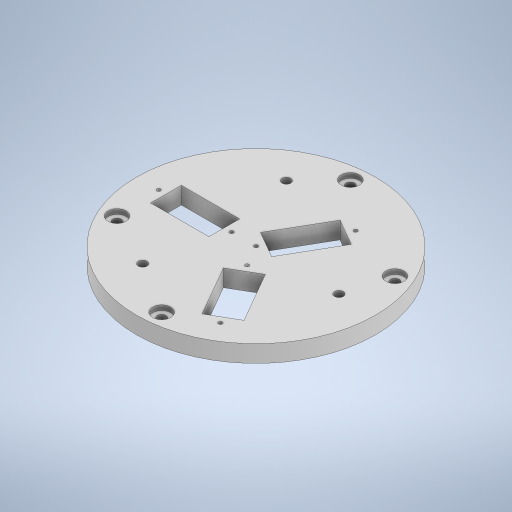
# Autodesk Inventor part: Servo Mounts
Saved by Autodesk Inventor 2023 (Build 270158000, 158)
## iProperties
Created: 2023-07-20
Part Number: Servo Mounts
Material: Generic
Document SubType Name: Modeling
Designer: campstudent
Density: 1 g/cm^3
Appearance: Default
Author: campstudent
Autodesk Inventor part; units mm, degrees
ref_plane "YZ Plane" through (0, 0, 0) normal (1, 0, 0) x (0, 1, 0)
ref_plane "XZ Plane" through (0, 0, 0) normal (0, 1, 0) x (-1, 0, 0)
ref_plane "XY Plane" through (0, 0, 0) normal (0, 0, 1) x (1, 0, 0)
sketch "Sketch1" plane through (0, 0, 0) normal (0, 1, 0) x (-1, 0, 0)
  circle A0 centre (0, 0) radius 45 construction
  line L0 (36.9, 6.3) -> (13, 6.3)
  line L1 (13, 6.3) -> (13, -6.3)
  line L2 (13, -6.3) -> (36.9, -6.3)
  line L3 (36.9, -6.3) -> (36.9, 6.3)
  line L4 (-12.994, 35.1063) -> (-23.906, 28.8063)
  line L5 (-23.906, 28.8063) -> (-11.956, 8.1083)
  line L6 (-1.044, 14.4083) -> (-12.994, 35.1063)
  line L7 (-11.956, 8.1083) -> (-1.044, 14.4083)
  line L8 (-18.9106, -20.1539) -> (-7.9987, -26.4539)
  line L9 (-7.9987, -26.4539) -> (3.9513, -5.7559)
  line L10 (-6.9606, 0.5441) -> (-18.9106, -20.1539)
  line L11 (3.9513, -5.7559) -> (-6.9606, 0.5441)
  circle A1 centre (11.0177, 0) radius 18 construction
  circle A2 centre (-5.5088, 9.5416) radius 18 construction
  circle A3 centre (-5.5088, -9.5416) radius 18 construction
  circle A4 centre (17, -29.4449) radius 1.8
  line L12 (0, 0) -> (20.2687, -35.1063)
  circle A5 centre (17, 29.4449) radius 1.8
  circle A6 centre (-34, 0) radius 1.8
  circle A7 centre (0, 0) radius 49
  line L13 (-5.5088, -9.5416) -> (-0.5088, -0.8813) construction
  line L14 (-5.5088, -9.5416) -> (4.4912, -9.5416) construction
  line L15 (-18.45, -31.9563) -> (3.4912, 6.0469) construction
  line L16 (-17.931, -18.4573) -> (-7.019, -24.7573) construction
  point P0 (-12.475, -21.6073)
  point P1 (-7.4794, -12.9547)
  dimension "d0" = 90
  dimension "d1" = 12.6
  dimension "d2" = 23.9
  dimension "d3" = 13
  dimension "d4" = 38.7
  dimension "d7" = 360
  dimension "d9" = 36
  dimension "d12" = 360
  dimension "d14" = 3.6
  dimension "d15" = 34
  dimension "d16" = -0.544
  dimension "d19" = 360
  dimension "d21" = 98
  dimension "d38" = 10
  dimension "d39" = 60
  dimension "d40" = 14.9588
  constraints: 34 end point, 7 centre point, 3 coincident, 2 horizontal, 2 midpoint, 2 parallel, 2 perpendicular, 2 point on line, 1 equal length, 26 other
  measures "d0" diameter of A0
  measures "d1" distance of L2.end L0.start
  measures "d2" distance of L0.start L0.end
  measures "d3" distance from line of point (0, 0) L1
  measures "d4" distance edge to line of A0 L2
  measures "d9" diameter of A1
  measures "d14" diameter of A4
  measures "d15" distance of A4.centre point (0, 0)
  measures "d16" distance from line of L12 L9.end
  measures "d21" diameter of A7
  measures "d38" distance of L13.start L13.end
  measures "d39" angle of L14 L13
  measures "d40" distance of point (0, 0) point (-7.479, -12.955)
extrude "Extrusion1" add sketch "Sketch1" along normal blind 7
sketch "Sketch2" plane through (0, 7, 0) normal (0, 1, 0) x (1, 0, 0)
  circle A0 centre (0, 0) radius 39.9 construction
  line L0 (1.044, -14.4083) -> (11.956, -8.1083) construction
  line L1 (6.5, -11.2583) -> (23.7787, -41.1859) construction
  circle A1 centre (19.95, -34.5544) radius 0.8
  circle A2 centre (14.95, 25.8942) radius 0.8
  circle A3 centre (-39.9, 0) radius 0.8
  line L2 (12.994, -35.1063) -> (1.044, -14.4083) construction
  line L3 (7.019, -24.7573) -> (17.931, -18.4573) construction
  line L4 (11.956, -8.1083) -> (23.906, -28.8063) construction
  circle A4 centre (5, -8.6603) radius 0.8
  circle A5 centre (0, 0) radius 0.8
  circle A6 centre (-10, 0) radius 0.8
  line L5 (0, 0) -> (22.1905, 38.4351) construction
  line L6 (0, 0) -> (44.3811, 0) construction
  line L7 (15.8257, 27.411) -> (10.8257, 18.7507)
  dimension "d24" = 79.8
  dimension "d25" = 1.6
  dimension "d28" = 360
  dimension "d34" = 360
  dimension "d41" = 60
  dimension "d42" = 10
  constraints: 10 end point, 6 centre point, 3 midpoint, 3 point on line, 2 coincident, 1 equal length, 1 horizontal, 1 perpendicular, 1 symmetric about line, 10 other
  measures "d25" diameter of A1
  measures "d41" angle of L6 L5
  measures "d42" distance of L7.start L7.end
extrude "Extrusion2" cut sketch "Sketch2" against normal through all
sketch "Sketch6" plane through (0, 7, 0) normal (0, 1, 0) x (1, 0, 0)
  line L0 (39.1506, 17.8109) -> (-4.1506, 42.8109)
  line L1 (-4.1506, 42.8109) -> (-39.1506, -17.8109)
  line L2 (-39.1506, -17.8109) -> (4.1506, -42.8109)
  line L3 (4.1506, -42.8109) -> (39.1506, 17.8109)
  line L4 (21.6506, -12.5) -> (-21.6506, 12.5) construction
  circle A0 centre (0, 0) radius 0.8 construction
  line L5 (0, 0) -> (-28.8675, 0) construction
  circle A1 centre (-39.1506, -17.8109) radius 1.8
  circle A2 centre (4.1506, -42.8109) radius 1.8
  circle A3 centre (-4.1506, 42.8109) radius 1.8
  circle A4 centre (39.1506, 17.8109) radius 1.8
  point P0 (0, 0)
  dimension "d43" = 25
  dimension "d44" = 25
  dimension "d45" = 35
  dimension "d46" = 35
  dimension "d47" = 30
  dimension "d48" = 3.6
  dimension "d49" = 3.6
  constraints: 12 end point, 4 centre point, 2 coincident, 2 midpoint, 2 parallel, 2 symmetric about line, 1 horizontal, 1 perpendicular, 1 point on line, 2 other
  measures "d43" distance from line of L1 point (0, 0)
  measures "d44" distance from line of L3 point (0, 0)
  measures "d45" distance from line of point (0, 0) L0
  measures "d46" distance from line of L2 point (0, 0)
  measures "d47" angle of L5 L4
  measures "d48" diameter of A1
  measures "d49" diameter of A2
extrude "Extrusion3" cut sketch "Sketch6" against normal through all contours L3 A4 L0 | L0 A4 L3 | A3 L1 L0 | L0 L1 A3 | A2 L2 L3 | L3 L2 A2 | A1 L2 L1 | L1 L2 A1
sketch "Sketch7" plane through (0, 7, 0) normal (0, 1, 0) x (1, 0, 0)
  circle A0 centre (-4.1506, 42.8109) radius 1.8 projected
  circle A1 centre (-4.1506, 42.8109) radius 3.75
  circle A2 centre (39.1506, 17.8109) radius 1.8 projected
  circle A3 centre (39.1506, 17.8109) radius 3.75
  circle A4 centre (-39.1506, -17.8109) radius 1.8 projected
  circle A5 centre (-39.1506, -17.8109) radius 3.75
  circle A6 centre (4.1506, -42.8109) radius 1.8 projected
  circle A7 centre (4.1506, -42.8109) radius 3.75
  point P0 (0, 0)
  dimension "d52" = 7.5
  dimension "d53" = 7.5
  dimension "d54" = 7.5
  dimension "d55" = 7.5
  constraints: 4 centre point, 4 coincident
  measures "d52" diameter of A1
  measures "d53" diameter of A3
  measures "d54" diameter of A5
  measures "d55" diameter of A7
extrude "Extrusion4" cut sketch "Sketch7" against normal blind 2 contours A0 | A1 | A2 | A3 | A5 | A6 | A7
body "Solid1"
